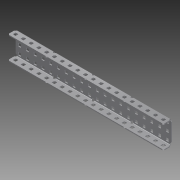
# Autodesk Inventor part: C-Channel 1x3x1x20 Hole
Saved by Autodesk Inventor 2016 (Build 200138000, 138)
## iProperties
Created: 2015-06-04
Part Number: C-Channel 1x3x1x20 Hole
Material: Aluminum 6061
Document SubType Name: Modeling
Designer: Martin
Density: 2.71 g/cm^3
Appearance: Aluminum - Polished
Mass: 102.48 g
Surface Area: 541.701 cm^2
Volume: 37.8155 cm^3
Author: Martin
Autodesk Inventor part; units mm, degrees
ref_plane "YZ Plane" through (0, 0, 0) normal (1, 0, 0) x (0, 1, 0)
ref_plane "XZ Plane" through (0, 0, 0) normal (0, 1, 0) x (-1, 0, 0)
ref_plane "XY Plane" through (0, 0, 0) normal (0, 0, 1) x (1, 0, 0)
sketch "Sketch1" plane through (0, 0, 0) normal (0, 1, 0) x (-1, 0, 0)
  line L0 (0, 0) -> (-444.5, 0)
  line L1 (-444.5, 0) -> (-444.5, -38.1)
  line L2 (-444.5, -38.1) -> (0, -38.1)
  line L3 (0, -38.1) -> (0, 0)
  dimension "d0" = 444.5
  dimension "d1" = 38.1
  constraints: 8 end point, 2 parallel, 1 horizontal, 1 perpendicular
  measures "d0" distance of L2.end L1.end
  measures "d1" distance of L1.end L0.end
extrude "Extrusion1" add sketch "Sketch1" along normal blind 1.6002
sketch "Sketch2" plane through (0, 1.6002, 0) normal (0, 1, 0) x (1, 0, 0)
  line L0 (0, 0) -> (444.5, 0) projected
  line L1 (444.5, 0) -> (444.5, 38.1) projected
  line L2 (444.5, 38.1) -> (0, 38.1) projected
  line L3 (0, 38.1) -> (0, 0) projected
  line L4 (0, 36.4998) -> (444.5, 36.4998)
  line L5 (0, 1.6002) -> (444.5, 1.6002)
  dimension "d4" = 1.6002
  dimension "d5" = 1.6002
  constraints: 4 end point, 4 point on line, 1 parallel, 1 perpendicular
  measures "d4" distance between parallel lines of L4 L2
  measures "d5" distance between parallel lines of L0 L5
extrude "Extrusion2" add sketch "Sketch2" along normal blind 12.7 contours L3 L5 L1 L0 | L3 L2 L1 L4
fillet "Fillet1" radius 0.8128 2 edges at (222.25, 1.6002, -36.4998) (222.25, 1.6002, -1.6002)
fillet "Fillet2" radius 2.413 2 edges at (222.25, 0, 0) (222.25, 0, -38.1)
sketch "Sketch3" plane through (0, 14.3002, 0) normal (0, 0, 1) x (1, 0, 0)
  line L0 (444.5, -11.8872) -> (444.5, 0) projected
  line L1 (0, 0) -> (444.5, 0) projected
  line L2 (442.8744, 0) -> (444.5, -1.6256)
  point P0 (0, -14.3002)
  dimension "d10" = 1.6256
  dimension "d11" = 1.6256
  constraints: 2 end point, 2 point on line
  measures "d10" distance of L2.end L0.end
  measures "d11" distance of L0.end L2.start
extrude "Extrusion3" cut sketch "Sketch3" against normal blind 3.175
pattern_linear "Rectangular Pattern1" count 5 spacing 63.5 along (-1, 0, 0) count 2 spacing 36.4998 along (0, 0, -1) of "Extrusion3"
sketch "Sketch4" plane through (0, 2.413, 0) normal (0, 0, 1) x (1, 0, 0)
  line L0 (0, 11.8872) -> (379.3744, 11.8872) projected
  line L1 (0, 0) -> (0, 11.8872) projected
  line L2 (127, 10.2616) -> (125.3744, 11.8872) projected
  line L3 (0, 10.2616) -> (1.6256, 11.8872)
  point P0 (61.8744, 11.8872)
  point P1 (0, -2.413)
  dimension "d20" = 1.6256
  dimension "d21" = 1.6256
  constraints: 2 end point, 2 point on line, 1 perpendicular
  measures "d20" distance of L0.start L3.end
  measures "d21" distance of L3.start L0.start
extrude "Extrusion4" cut sketch "Sketch4" against normal blind 3.175
pattern_linear "Rectangular Pattern2" count 7 spacing 63.5 along (1, 0, 0) count 2 spacing 36.4998 along (0, 0, -1) of "Extrusion4"
sketch "Sketch5" plane through (0, 2.413, 0) normal (0, 0, 1) x (1, 0, 0)
  line L0 (444.5, 0) -> (0, 0) projected
  line L1 (444.5, 0) -> (444.5, 10.2616) projected
  line L2 (444.5, 10.2616) -> (442.8744, 11.8872) projected
  line L3 (0, -2.413) -> (444.5, -2.413) projected
  line L4 (444.5, 1.6256) -> (442.8744, 0)
  line L5 (442.8744, 0) -> (444.5, 0)
  line L6 (444.5, 1.6256) -> (446.1256, 0)
  line L7 (446.1256, 0) -> (444.5, 0)
  line L8 (0, -0.8128) -> (444.5, -0.8128) projected
  line L9 (441.8111, -2.413) -> (442.8744, 0)
  line L10 (441.8111, -2.413) -> (444.5, -2.413)
  line L11 (447.1889, -2.413) -> (446.1256, 0)
  line L12 (447.1889, -2.413) -> (444.5, -2.413)
  dimension "d30" = 1.6256
  constraints: 16 end point, 3 point on line, 2 parallel, 2 symmetric about line, 1 perpendicular
  measures "d30" distance of L0.start L4.start
revolve "Revolution1" cut sketch "Sketch5" angle 360 about axis through (0, 0, 0) along (1, 0, 0)
pattern_linear "Rectangular Pattern3" count 5 spacing 63.5 along (-1, 0, 0) count 2 spacing 36.4998 along (0, 0, -1) of "Revolution1"
sketch "Sketch6" plane through (1.6256, 14.3002, 0) normal (0, 0, 1) x (1, 0, 0)
  line L0 (442.8744, -10.2616) -> (442.8744, -1.6256) projected
  line L1 (254, 0) -> (441.2488, 0) projected
  line L2 (434.721, -3.937) -> (438.3278, -3.937)
  line L3 (438.8358, -4.445) -> (438.8358, -8.0518)
  line L4 (438.3278, -8.5598) -> (434.721, -8.5598)
  line L5 (434.213, -8.0518) -> (434.213, -4.445)
  arc A0 (434.721, -3.937) -> (434.213, -4.445) centre (434.721, -4.445) ccw
  arc A1 (438.8358, -4.445) -> (438.3278, -3.937) centre (438.3278, -4.445) ccw
  arc A2 (438.3278, -8.5598) -> (438.8358, -8.0518) centre (438.3278, -8.0518) ccw
  arc A3 (434.213, -8.0518) -> (434.721, -8.5598) centre (434.721, -8.0518) ccw
  point P0 (381, 0)
  point P1 (-1.6256, -14.3002)
  point P2 (438.8358, -8.5598)
  point P3 (438.8358, -3.937)
  point P4 (434.213, -8.5598)
  dimension "d38" = 4.6228
  dimension "d39" = 4.6228
  dimension "d40" = 3.937
  dimension "d41" = 4.0386
  dimension "d42" = 0.508
  constraints: 8 end point, 8 point on circle, 8 tangent, 6 point on line, 4 centre point, 3 equal radius, 2 parallel, 1 horizontal, 1 perpendicular
  measures "d38" distance of point (438.836, -8.56) point (434.213, -8.56)
  measures "d39" distance of point (438.836, -3.937) point (438.836, -8.56)
  measures "d40" distance between parallel lines of L1 L2
  measures "d41" distance between parallel lines of L0 L3
  measures "d42" radius of A0
extrude "Extrusion5" cut sketch "Sketch6" against normal blind 61.9125
pattern_linear "Rectangular Pattern4" count 20 spacing 12.7 along (-1, 0, 0) of "Extrusion5"
sketch "Sketch7" plane through (0, 0, 0) normal (0, -1, 0) x (1, 0, 0)
  line L0 (444.5, -4.0386) -> (444.5, -32.4612) projected
  line L1 (436.3466, -29.4386) -> (439.9534, -29.4386)
  line L2 (440.4614, -29.9466) -> (440.4614, -33.5534)
  line L3 (439.9534, -34.0614) -> (436.3466, -34.0614)
  line L4 (435.8386, -33.5534) -> (435.8386, -29.9466)
  line L5 (382.1432, -38.1) -> (443.3568, -38.1) projected
  arc A0 (436.3466, -29.4386) -> (435.8386, -29.9466) centre (436.3466, -29.9466) ccw
  arc A1 (439.9534, -34.0614) -> (440.4614, -33.5534) centre (439.9534, -33.5534) ccw
  arc A2 (440.4614, -29.9466) -> (439.9534, -29.4386) centre (439.9534, -29.9466) ccw
  arc A3 (435.8386, -33.5534) -> (436.3466, -34.0614) centre (436.3466, -33.5534) ccw
  point P0 (0, 0)
  point P1 (440.4614, -34.0614)
  point P2 (440.4614, -29.4386)
  point P3 (435.8386, -34.0614)
  dimension "d48" = 4.6228
  dimension "d49" = 4.6228
  dimension "d50" = 4.0386
  dimension "d51" = 4.0386
  dimension "d52" = 0.508
  constraints: 8 end point, 8 point on circle, 8 tangent, 6 point on line, 4 centre point, 3 equal radius, 2 parallel, 1 horizontal, 1 perpendicular
  measures "d48" distance of point (440.461, -34.061) point (435.839, -34.061)
  measures "d49" distance of point (440.461, -29.439) point (440.461, -34.061)
  measures "d50" distance between parallel lines of L0 L2
  measures "d51" distance between parallel lines of L5 L3
  measures "d52" radius of A0
extrude "Extrusion6" cut sketch "Sketch7" against normal blind 15.875
pattern_linear "Rectangular Pattern5" count 20 spacing 12.7 along (-1, 0, 0) count 3 spacing 12.7 along (0, 0, 1) of "Extrusion6"
sketch "Sketch8" plane through (1.6256, 14.3002, 0) normal (0, 0, 1) x (1, 0, 0)
  line L0 (434.721, -3.937) -> (438.3278, -3.937) projected
  line L1 (438.8358, -4.445) -> (438.8358, -8.0518) projected
  circle A0 centre (436.5244, -6.2484) radius 2.3114
  point P0 (-1.6256, -14.3002)
  dimension "d61" = 4.6228
  constraints: 2 tangent, 1 centre point
  measures "d61" diameter of A0
surface extrude "ExtrusionSrf1" sketch "Sketch8" against normal blind 1.6002 shown no curves A0
pattern_linear "Rectangular Pattern6" count 20 spacing 12.7 along (-1, 0, 0) count 2 spacing 36.4998 along (0, 0, -1) of "ExtrusionSrf1"
sketch "Sketch9" plane through (0, 0, 0) normal (0, -1, 0) x (1, 0, 0)
  line L0 (436.3466, -4.0386) -> (439.9534, -4.0386) projected
  line L1 (435.8386, -8.1534) -> (435.8386, -4.5466) projected
  circle A0 centre (438.15, -6.35) radius 2.3114
  point P0 (0, 0)
  dimension "d70" = 4.6228
  constraints: 2 tangent, 1 centre point
  measures "d70" diameter of A0
surface extrude "ExtrusionSrf71" sketch "Sketch9" against normal blind 1.6002 shown no curves A0
pattern_linear "Rectangular Pattern8" count 20 spacing 12.7 along (-1, 0, 0) count 3 spacing 12.7 along (0, 0, -1) of "ExtrusionSrf71"
sketch "Sketch11" plane through (0, 14.3002, 0) normal (0, 1, 0) x (1, 0, 0)
  line L0 (0, 0) -> (190.5, 0)
  line L1 (190.5, 0) -> (190.5, 38.1)
  line L2 (190.5, 38.1) -> (0, 38.1)
  line L3 (0, 38.1) -> (0, 0)
  point P0 (63.5, 38.1)
  point P1 (127, 0)
  dimension "d441" = 190.5
  dimension "d442" = 38.1
  constraints: 8 end point, 2 parallel, 1 horizontal, 1 perpendicular
  measures "d441" distance of L2.end L1.end
  measures "d442" distance of L1.end L0.end
extrude "Extrusion7" cut sketch "Sketch11" against normal through all
body "Solid1"
body "Srf1"
body "Srf2"
body "Srf3"
body "Srf4"
body "Srf5"
body "Srf6"
body "Srf7"
body "Srf8"
body "Srf9"
body "Srf10"
body "Srf11"
body "Srf12"
body "Srf13"
body "Srf14"
body "Srf15"
body "Srf16"
body "Srf17"
body "Srf18"
body "Srf19"
body "Srf20"
body "Srf36"
body "Srf37"
body "Srf38"
body "Srf39"
body "Srf40"
body "Srf41"
body "Srf42"
body "Srf43"
body "Srf44"
body "Srf45"
body "Srf46"
body "Srf47"
body "Srf48"
body "Srf49"
body "Srf50"
body "Srf51"
body "Srf52"
body "Srf53"
body "Srf54"
body "Srf55"
body "Srf71"
body "Srf176"
body "Srf177"
body "Srf178"
body "Srf179"
body "Srf180"
body "Srf181"
body "Srf182"
body "Srf183"
body "Srf184"
body "Srf185"
body "Srf186"
body "Srf187"
body "Srf188"
body "Srf189"
body "Srf190"
body "Srf191"
body "Srf192"
body "Srf193"
body "Srf194"
body "Srf210"
body "Srf211"
body "Srf212"
body "Srf213"
body "Srf214"
body "Srf215"
body "Srf216"
body "Srf217"
body "Srf218"
body "Srf219"
body "Srf220"
body "Srf221"
body "Srf222"
body "Srf223"
body "Srf224"
body "Srf225"
body "Srf226"
body "Srf227"
body "Srf228"
body "Srf229"
body "Srf245"
body "Srf246"
body "Srf247"
body "Srf248"
body "Srf249"
body "Srf250"
body "Srf251"
body "Srf252"
body "Srf253"
body "Srf254"
body "Srf255"
body "Srf256"
body "Srf257"
body "Srf258"
body "Srf259"
body "Srf260"
body "Srf261"
body "Srf262"
body "Srf263"
body "Srf264"
